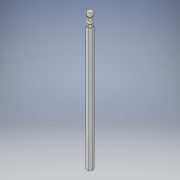
# Autodesk Inventor part: pencil (unsharpened)
Saved by Autodesk Inventor 2017 (Build 210142000, 142)
## iProperties
Created: 2018-03-26
Part Number: pencil (unsharpened)
Material: Generic
Document SubType Name: Modeling
Designer: Braxton
Density: 1 g/cm^3
Appearance: Default
Author: Braxton
Autodesk Inventor part; units mm, degrees
ref_plane "YZ Plane" through (0, 0, 0) normal (1, 0, 0) x (0, 1, 0)
ref_plane "XZ Plane" through (0, 0, 0) normal (0, 1, 0) x (-1, 0, 0)
ref_plane "XY Plane" through (0, 0, 0) normal (0, 0, 1) x (1, 0, 0)
sketch "Sketch1" plane through (0, 0, 0) normal (0, 1, 0) x (-1, 0, 0)
  line L0 (0.1683, 0.2916) -> (0.3367, 0)
  line L1 (0.3367, 0) -> (0.1683, -0.2916)
  line L2 (0.1683, -0.2916) -> (-0.1683, -0.2916)
  line L3 (-0.1683, -0.2916) -> (-0.3367, 0)
  line L4 (-0.3367, 0) -> (-0.1683, 0.2916)
  line L5 (-0.1683, 0.2916) -> (0.1683, 0.2916)
  point P0 (0, 0)
  point P1 (0, 0)
  dimension "d0" = 0.5831
  constraints: 12 end point, 1 coincident, 1 horizontal, 13 other
  measures "d0" distance between parallel lines of L2 L5
extrude "wooden part of pencil" add sketch "Sketch1" along normal blind 14.1669
sketch "Sketch3" plane through (0, 0, 0) normal (0, 0, 1) x (1, 0, 0)
  line L0 (-0.1683, 14.1669) -> (0.1683, 14.1669) projected
  line L1 (0, 14.1669) -> (0, 15.2326)
  line L2 (0, 14.1669) -> (-0.3106, 14.1669)
  line L3 (-0.3106, 14.1669) -> (-0.3106, 14.2388)
  line L4 (-0.3111, 14.537) -> (-0.3111, 14.8651)
  line L5 (-0.3106, 15.1659) -> (-0.3106, 15.2326)
  line L6 (-0.3106, 15.2326) -> (0, 15.2326)
  line L7 (-0.3106, 14.2875) -> (-0.262, 14.2875) construction
  line L8 (-0.3106, 14.3552) -> (-0.262, 14.3552) construction
  line L9 (-0.3106, 14.423) -> (-0.262, 14.423) construction
  line L10 (-0.3106, 14.4907) -> (-0.262, 14.4907) construction
  line L11 (-0.3106, 14.914) -> (-0.262, 14.914) construction
  line L12 (-0.3111, 14.9818) -> (-0.2624, 14.9818) construction
  line L13 (-0.3106, 15.0495) -> (-0.262, 15.0495) construction
  line L14 (-0.3106, 15.1172) -> (-0.262, 15.1172) construction
  arc A0 (-0.2874, 14.3551) -> (-0.2764, 14.2853) centre (-0.2745, 14.3214) ccw
  arc A1 (-0.2863, 14.423) -> (-0.2874, 14.3551) centre (-0.2745, 14.3888) ccw
  arc A2 (-0.2824, 14.4923) -> (-0.2863, 14.423) centre (-0.2745, 14.4571) ccw
  arc A3 (-0.2871, 14.9818) -> (-0.2765, 14.9119) centre (-0.2745, 14.948) ccw
  arc A4 (-0.2871, 15.0495) -> (-0.2871, 14.9818) centre (-0.2745, 15.0157) ccw
  arc A5 (-0.2764, 15.1194) -> (-0.2871, 15.0495) centre (-0.2745, 15.0834) ccw
  arc A6 (-0.2764, 14.2853) -> (-0.3106, 14.2388) centre (-0.262, 14.2388) ccw
  line L15 (-0.262, 14.2388) -> (-0.262, 15.1172) construction
  arc A7 (-0.3111, 14.537) -> (-0.2824, 14.4923) centre (-0.262, 14.537) ccw
  arc A8 (-0.2765, 14.9119) -> (-0.3111, 14.8651) centre (-0.262, 14.8651) ccw
  arc A9 (-0.3106, 15.1659) -> (-0.2764, 15.1194) centre (-0.262, 15.1659) ccw
  line L16 (-0.262, 15.1172) -> (-0.262, 15.1749) construction
  line L17 (-0.2745, 14.3888) -> (-0.2745, 14.423)
  line L18 (-0.2745, 14.4571) -> (-0.2745, 14.423)
  line L19 (-0.2745, 14.3888) -> (-0.2745, 14.3552)
  line L20 (-0.2745, 14.3214) -> (-0.2745, 14.3552)
  point P0 (0, 0)
  dimension "d3" = 0.3106
  dimension "d4" = 0.1206
  dimension "d10" = 0.0487
  dimension "d13" = 0.0677
  dimension "d14" = 0.4233
  dimension "d15" = 0.1154
  dimension "d16" = 0.0487
  dimension "d17" = 0.072
  dimension "d18" = 0.0361
  dimension "d20" = 0.0339
  dimension "d21" = 0.0126
  dimension "d22" = 0.0677
  dimension "d23" = 0.0677
  dimension "d24" = 0.0677
  dimension "d25" = 0.0677
  dimension "d26" = 0.0677
  dimension "d27" = 0.0491
  dimension "d28" = 0.0463
  dimension "d29" = 0.049
  constraints: 40 end point, 20 point on circle, 10 centre point, 10 point on line, 9 horizontal, 7 parallel, 6 vertical, 5 equal radius, 4 tangent, 3 perpendicular, 2 collinear, 2 midpoint
  measures "d3" distance of L1.start L2.end
  measures "d4" distance of L2.end L7.start
  measures "d10" distance of L7.start L7.end
  measures "d13" distance between parallel lines of L8 L7
  measures "d14" distance between parallel lines of L10 L11
  measures "d15" distance between parallel lines of L6 L14
  measures "d16" radius of A6
  measures "d17" distance of L2.end L3.end
  measures "d18" radius of A0
  measures "d20" distance from line of L7 L20.start
  measures "d21" distance from line of L15 L20.start
  measures "d22" distance between parallel lines of L9 L8
  measures "d23" distance between parallel lines of L10 L9
  measures "d24" distance between parallel lines of L12 L11
  measures "d25" distance between parallel lines of L13 L12
  measures "d26" distance between parallel lines of L14 L13
  measures "d27" radius of A7
  measures "d28" distance from line of L10 A7.centre
  measures "d29" distance from line of L11 A8.centre
revolve "connection for pencil and eraser" add sketch "Sketch3" angle 360 about axis through (0, 14.1669, 0) along (0, 1, 0)
sketch "Sketch4" plane through (0, 0, 0) normal (0, 0, 1) x (1, 0, 0)
  line L0 (0.3106, 15.2326) -> (-0.3106, 15.2326) projected
  line L1 (0, 15.2326) -> (-0.2799, 15.2326)
  line L2 (-0.2799, 15.2326) -> (-0.2799, 15.6231)
  line L3 (-0.2799, 15.6231) -> (0, 15.6231)
  line L4 (0, 15.6231) -> (0, 15.2326)
  point P0 (0, 0)
  dimension "d31" = 0.2799
  dimension "d32" = 0.3905
  constraints: 8 end point, 3 perpendicular, 1 midpoint, 1 point on line
  measures "d31" distance of L1.start L1.end
  measures "d32" distance of L1.end L2.end
revolve "eraser" add sketch "Sketch4" angle 360 about axis through (0, 15.6231, 0) along (0, -1, 0)
equation "\"d22\" = d13"
equation "\"d23\" = d13"
equation "\"d24\" = d13"
equation "\"d25\" = d13"
equation "\"d26\" = d13"
body "Solid1"
